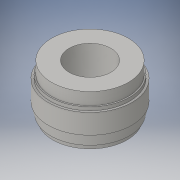
# Autodesk Inventor part: 50mm_1_4G_body_disassembled
Saved by Autodesk Inventor 2016 (Build 200138000, 138)
## iProperties
Created: 2016-08-10
Part Number: 50mm_1_4G_body_disassembled
Material: Iron, Cast
Document SubType Name: Modeling
Designer: voigt
Density: 7.15 g/cm^3
Appearance: Iron Gray
Author: voigt
Autodesk Inventor part; units mm, degrees
ref_plane "YZ Plane" through (0, 0, 0) normal (1, 0, 0) x (0, 1, 0)
ref_plane "XZ Plane" through (0, 0, 0) normal (0, 1, 0) x (-1, 0, 0)
ref_plane "XY Plane" through (0, 0, 0) normal (0, 0, 1) x (1, 0, 0)
sketch "Sketch1" plane through (0, 0, 0) normal (1, 0, 0) x (0, 1, 0)
  line L0 (0, -8.868) -> (0, 53.208) construction
  line L1 (-7.2, 0) -> (43.2, 0) construction
  line L2 (0, 0) -> (29, 0)
  line L3 (29, 0) -> (29, 0.84)
  line L4 (29, 0.84) -> (32, 0.84)
  line L5 (32, 0.84) -> (33.85, 4.84)
  line L6 (33.85, 4.84) -> (36, 13.84)
  line L7 (36, 13.84) -> (36, 30.84)
  line L8 (36, 30.84) -> (34.15, 30.84)
  line L9 (34.15, 30.84) -> (34.15, 33.84)
  line L10 (34.15, 33.84) -> (33, 33.84)
  line L11 (33, 33.84) -> (33, 44.34)
  line L12 (33, 44.34) -> (0, 44.34)
  line L13 (0, 44.34) -> (0, 0)
  dimension "d2" = 58
  dimension "d3" = 0.84
  dimension "d5" = 64
  dimension "d6" = 4
  dimension "d7" = 67.7
  dimension "d8" = 72
  dimension "d9" = 9
  dimension "d10" = 17
  dimension "d11" = 3
  dimension "d12" = 68.3
  dimension "d13" = 10.5
  dimension "d14" = 66
  constraints: 24 end point, 4 perpendicular, 3 horizontal, 2 collinear, 2 point on line, 2 vertical
  measures "d2" diameter of L2.end L0
  measures "d3" distance of L2.end L3.end
  measures "d5" diameter of L4.end L0
  measures "d6" distance from line of L4 L5.end
  measures "d7" diameter of L5.end L0
  measures "d8" diameter of L6.end L0
  measures "d9" vertical distance of L5.end L6.end
  measures "d10" distance of L6.end L7.end
  measures "d11" distance of L8.end L9.end
  measures "d12" diameter of L9 L0
  measures "d13" distance of L10.end L11.end
  measures "d14" diameter of L11 L0
revolve "Revolution1" add sketch "Sketch1" angle 360 about axis through (0, 0, -10) along (0, 0, 1)
sketch "Sketch4" plane through (0, 0, 44.34) normal (0, 0, 1) x (1, 0, 0)
  circle A0 centre (0, 0) radius 18
  dimension "d19" = 36
  constraints: 1 centre point, 1 coincident
  measures "d19" diameter of A0
extrude "Extrusion1" cut sketch "Sketch4" against normal up to next
body "Solid1"
